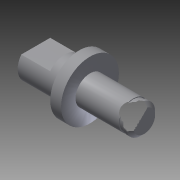
# Autodesk Inventor part: 13_1087_016
Saved by Autodesk Inventor 2014 (Build 180170000, 170)
## iProperties
Created: 2013-09-03
Part Number: 13_1087_016
Material: Allgemein
Document SubType Name: Modeling
Designer: vogel
Density: 1 g/cm^3
Appearance: Vorgabe
Author: vogel
Autodesk Inventor part; units mm, degrees
ref_plane "YZ Plane" through (0, 0, 0) normal (1, 0, 0) x (0, 1, 0)
ref_plane "XZ Plane" through (0, 0, 0) normal (0, 1, 0) x (-1, 0, 0)
ref_plane "XY Plane" through (0, 0, 0) normal (0, 0, 1) x (1, 0, 0)
sketch "Skizze1" plane through (0, 0, 0) normal (0, 0, 1) x (1, 0, 0)
  line L0 (-18, 0) -> (3, 0) projected
  line L1 (0, -0.8) -> (0, 4.8) projected
  line L2 (0, 2) -> (-7.5, 2)
  line L3 (-7.5, 2) -> (-7.5, 4)
  line L4 (-7.5, 4) -> (-9, 4)
  line L5 (-9, 4) -> (-9, 2.5)
  line L6 (-9, 2.5) -> (-15, 2.5)
  line L7 (-15, 2.5) -> (-15, 0)
  line L8 (-15, 0) -> (0, 0)
  line L9 (0, 0) -> (0, 2)
  dimension "d0" = 4
  dimension "d1" = 8
  dimension "d2" = 5
  dimension "d3" = 7.5
  dimension "d4" = 1.5
  dimension "d5" = 6
  constraints: 16 end point, 3 parallel, 3 perpendicular, 2 collinear, 1 midpoint, 1 point on line
  measures "d0" diameter of L2 L0
  measures "d1" diameter of L4 L0
  measures "d2" diameter of L6 L0
  measures "d3" distance of L2.start L2.end
  measures "d4" distance of L3.end L4.end
  measures "d5" distance of L5.end L6.end
revolve "Umdrehung1" add sketch "Skizze1" angle 360 about axis through (-10, 0, 0) along (1, 0, 0)
sketch "Skizze2" plane through (-15, 0, 0) normal (-1, 0, 0) x (0, 0, 1)
  circle A0 centre (0, 0) radius 2.5 projected
  line L0 (1.5, 2) -> (1.5, -2)
  dimension "d7" = 1
  constraints: 2 end point, 2 point on circle, 1 vertical
  measures "d7" distance edge to line of A0 L0
extrude "Extrusion1" cut sketch "Skizze2" against normal blind 4 contours A0 L0 picked at (1.6398, 0.534)
sketch "Skizze3" plane through (0, 0, 0) normal (0, 1, 0) x (-1, 0, 0)
  line L0 (1.5, 2) -> (1, 2)
  line L1 (1, 2) -> (1, 1.9)
  line L2 (1, 1.9) -> (1.5, 1.9)
  line L3 (1.5, 1.9) -> (1.5, 2)
  line L4 (2.4, 0) -> (-0.4, 0) projected
  line L5 (0, -0.4) -> (0, 2.4) projected
  point P0 (0, 0)
  dimension "d10" = 3.8
  dimension "d11" = 1.5
  dimension "d12" = 0.5
  dimension "d13" = 4
  constraints: 8 end point, 2 parallel, 1 horizontal, 1 perpendicular
  measures "d10" diameter of L2 L4
  measures "d11" distance between parallel lines of L3 L5
  measures "d12" distance between parallel lines of L1 L3
  measures "d13" diameter of L0 L4
revolve "Umdrehung2" cut sketch "Skizze3" angle 360 about axis through (-10, 0, 0) along (1, 0, 0)
chamfer "Fase1" distance 0.5 angle 45 1 edges at (0, -2, 0)
